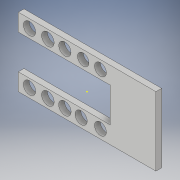
# Autodesk Inventor part: Back Slide plate
Saved by Autodesk Inventor 2017 (Build 210142000, 142)
## iProperties
Created: 2017-10-11
Part Number: Back Slide plate
Material: Generic
Document SubType Name: Modeling
Designer: Kenneth
Density: 1 g/cm^3
Appearance: Default
Author: Kenneth
Autodesk Inventor part; units mm, degrees
ref_plane "YZ Plane" through (0, 0, 0) normal (1, 0, 0) x (0, 1, 0)
ref_plane "XZ Plane" through (0, 0, 0) normal (0, 1, 0) x (-1, 0, 0)
ref_plane "XY Plane" through (0, 0, 0) normal (0, 0, 1) x (1, 0, 0)
sketch "Sketch1" plane through (0, 0, 0) normal (0, 0, 1) x (1, 0, 0)
  line L0 (-76.2, -38.1) -> (76.2, -38.1)
  line L1 (76.2, -38.1) -> (76.2, 38.1)
  line L2 (76.2, 38.1) -> (-76.2, 38.1)
  line L3 (-76.2, 38.1) -> (-76.2, -38.1)
  line L4 (-76.2, -38.1) -> (76.2, 38.1) construction
  line L5 (76.2, -38.1) -> (-76.2, 38.1) construction
  point P0 (0, 0)
  dimension "d0" = 152.4
  dimension "d1" = 76.2
  constraints: 12 end point, 2 midpoint, 2 parallel, 1 horizontal, 1 perpendicular
  measures "d0" distance of L1.end L2.end
  measures "d1" distance of L0.end L1.end
extrude "Extrusion1" add sketch "Sketch1" along normal blind 6.35
sketch "Sketch2" plane through (0, 0, 6.35) normal (0, 0, 1) x (1, 0, 0)
  line L0 (-177.8, -19.05) -> (25.4, -19.05)
  line L1 (25.4, -19.05) -> (25.4, 19.05)
  line L2 (25.4, 19.05) -> (-177.8, 19.05)
  line L3 (-177.8, 19.05) -> (-177.8, -19.05)
  line L4 (-76.2, 38.1) -> (-76.2, -38.1) projected
  line L5 (-177.8, -19.05) -> (25.4, 19.05) construction
  line L6 (25.4, -19.05) -> (-177.8, 19.05) construction
  point P0 (0, 0)
  point P1 (-76.2, 0)
  dimension "d4" = 203.2
  dimension "d5" = 38.1
  constraints: 12 end point, 3 midpoint, 2 parallel, 1 horizontal, 1 perpendicular
  measures "d4" distance of L1.end L2.end
  measures "d5" distance of L0.end L1.end
extrude "Extrusion2" cut sketch "Sketch2" against normal blind 6.35
sketch "Sketch3" plane through (0, 0, 6.35) normal (0, 0, 1) x (1, 0, 0)
  circle A0 centre (-63.7658, 28.7049) radius 6.8157
  circle A1 centre (-43.4673, 28.7049) radius 6.9621
  circle A2 centre (-24.6042, 28.7049) radius 6.7661
  circle A3 centre (-4.3057, 28.7049) radius 6.3561
  circle A4 centre (14.7625, 28.7049) radius 6.5611
  circle A5 centre (-63.7658, -28.1923) radius 6.8434
  circle A6 centre (-43.4673, -28.1923) radius 6.9621
  circle A7 centre (-24.6042, -28.1923) radius 6.8771
  circle A8 centre (-6.6217, -28.1923) radius 6.735
  circle A9 centre (14.7625, -28.1923) radius 6.5611
  point P0 (0, 0)
  dimension "d8" = 13.6313
  constraints: 10 centre point
  measures "d8" diameter of A0
extrude "Extrusion3" cut sketch "Sketch3" against normal blind 6.35
sketch "Sketch4" plane through (0, 0, 6.35) normal (0, 0, 1) x (1, 0, 0)
  point P0 (0, 0)
body "Solid1"
